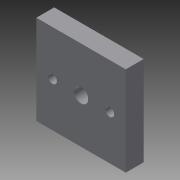
# Autodesk Inventor part: shf8gen
Saved by Autodesk Inventor 2014 (Build 180170000, 170)
## iProperties
Created: 2014-07-13
Part Number: shf8gen
Material: Generic
Document SubType Name: Modeling
Designer: cruiser
Density: 1 g/cm^3
Appearance: Default
Author: cruiser
Autodesk Inventor part; units mm, degrees
ref_plane "YZ Plane" through (0, 0, 0) normal (1, 0, 0) x (0, 1, 0)
ref_plane "XZ Plane" through (0, 0, 0) normal (0, 1, 0) x (-1, 0, 0)
ref_plane "XY Plane" through (0, 0, 0) normal (0, 0, 1) x (1, 0, 0)
sketch "Sketch4" plane through (0, 0, 0) normal (0, 1, 0) x (-1, 0, 0)
  line L0 (25, -25) -> (-25, -25)
  line L1 (-25, -25) -> (-25, 25)
  line L2 (-25, 25) -> (25, 25)
  line L3 (25, 25) -> (25, -25)
  line L4 (25, -25) -> (-25, 25) construction
  line L5 (-25, -25) -> (25, 25) construction
  point P0 (0, 0)
  dimension "d18" = 50
  dimension "d19" = 50
  constraints: 12 end point, 2 midpoint, 2 parallel, 1 horizontal, 1 perpendicular
  measures "d18" distance of L1.end L2.end
  measures "d19" distance of L0.end L1.end
extrude "Extrusion4" add sketch "Sketch4" along normal blind 10
sketch "Sketch5" plane through (0, 10, 0) normal (0, 1, 0) x (1, 0, 0)
  circle A0 centre (0, 0) radius 4
  circle A1 centre (-16, 0) radius 2.5
  circle A2 centre (16, 0) radius 2.5
  line L0 (16, -15) -> (-16, -15)
  line L1 (-16, -15) -> (-16, 15)
  line L2 (-16, 15) -> (16, 15)
  line L3 (16, 15) -> (16, -15)
  line L4 (16, -15) -> (-16, 15) construction
  line L5 (-16, -15) -> (16, 15) construction
  line L6 (-16, 0) -> (0, 0)
  dimension "d22" = 8
  dimension "d23" = 5
  dimension "d27" = 360
  dimension "d31" = 32
  dimension "d32" = 30
  constraints: 14 end point, 3 centre point, 3 midpoint, 2 coincident, 2 parallel, 2 perpendicular, 1 horizontal, 5 other
  measures "d22" diameter of A0
  measures "d23" diameter of A1
  measures "d31" distance of L1.end L2.end
  measures "d32" distance of L0.end L1.end
extrude "shf8 holes" cut sketch "Sketch5" against normal up to next contours A0 | A1 L1 L6 | L6 L1 A1 | L1 A1 | L3 A2 | A2 L3
equation "\"d22\" = shaft_hole"
equation "\"d23\" = mount_hole"
equation "\"d31\" = 2 * hole_spacing"
equation "\"hole_spacing\" = 16"
equation "\"shaft_hole\" = 8"
equation "\"mount_hole\" = 5"
body "Solid2"
